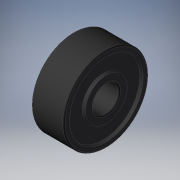
# Autodesk Inventor part: B624ZZ
Saved by Autodesk Inventor 2019 (Build 230136000, 136)
## iProperties
Created: 2024-10-07
Part Number: B624ZZ
Material: Generic
Catalog Web Link: www.cadenas.de
Description: B6 _ _ ZZ, B6 _ _ AZZ, SB6 _ _ ZZ, SB6 _ _ AZZ, BR _ _ ZZ, SBR _ _ ZZ-Small Ball Bearings - Double Shield Type
Vendor: MISUMI
Document SubType Name: Modeling
Designer: psAdmin
Manufacturer: MISUMI
Mass: 0.528594 g
Surface Area: 5.56418 cm^2
Volume: 0.528594 cm^3
Density: 1 g/cm^3
Appearance: PSOLRGB-175-175-175
Category: PARTsolutions
Company: MISUMI
Title: B624ZZ
Author: Cadenas PARTsolutions
Comments: Small Ball Bearings - Double Shield Type
PSOL_IDENT_0: {$CADENAS_DATA/23d-libs/misumi/metric/12_bearing_holders/sb685zz.prj},218 {VTYP=3D},{NB=B624ZZ},{LIN
PSOL_IDENT_1: A=B624ZZ},{NN=B6 _ _ ZZ, B6 _ _ AZZ, SB6 _ _ ZZ, SB6 _ _ AZZ, BR _ _ ZZ, SBR _ _ ZZ},{DATE=30.06.202
PSOL_IDENT_2: 1 12:59:24},{GEOMDATE=23.07.2013 00:00:00},{VERSION=},{LINEID=60},{WBVAR=MAT},{WBNUMERIC=}  {NB=B624
PSOL_IDENT_3: ZZ},{LINA=B624ZZ},{KT=DUMMY},{PN=B624ZZ},{MAT=},{BN=624ZZ},{DD=4.0},{A=3.9530},{BB=0.850},{C=1.200},
PSOL_IDENT_4: {D=13},{B=5.0},{RR=0.20},{CR=1310},{COR=490},{CRS=1310},{CRSS=1106},{CORS=490},{CORSS=390},{DS=5.60}
PSOL_IDENT_5: ,{DDHH=11.40},{R=0.20},{MASS=3.2},{X=0},{BN2=B624ZZ}
NB: B624ZZ
NN: B6 _ _ ZZ, B6 _ _ AZZ, SB6 _ _ ZZ, SB6 _ _ AZZ, BR _ _ ZZ, SBR _ _ ZZ
NT: Small Ball Bearings - Double Shield Type
NBSYN: $PN.
LINA: B624ZZ
CATALOG: Misumi
PN: B624ZZ
MAT: 52100 Bearing Steel
BN: 624ZZ
DD: 4
D: 13
B: 5
RR: 0.2
CR: 1310
COR: 490
DS: 5.6
DDHH: 11.4
R: 0.2
MASS: 3.2
X: 0
SUPPLIER: MISUMI
ARTICLENO: B624ZZ
BOMINFO: B624ZZ
CREATOR: CADENAS GmbH
Autodesk Inventor part; units mm, degrees
sketch "Sketch_1" plane through (0, 0, 0) normal (0, 0, 1) x (1, 0, 0)
  line L0 (4.8, 0) -> (0.2, 0)
  arc A0 (0, 2.2) -> (0.2, 2) centre (0.2, 2.2) ccw
  line L1 (0.2, 2) -> (4.8, 2)
  arc A1 (4.8, 2) -> (5, 2.2) centre (4.8, 2.2) ccw
  line L2 (5, 2.2) -> (5, 3.2)
  line L3 (5, 3.2) -> (4.4765, 3.2)
  line L4 (4.4765, 3.2) -> (4.4765, 5.65)
  line L5 (4.4765, 5.65) -> (5, 5.65)
  line L6 (5, 5.65) -> (5, 6.3)
  arc A2 (5, 6.3) -> (4.8, 6.5) centre (4.8, 6.3) ccw
  line L7 (4.8, 6.5) -> (0.2, 6.5)
  arc A3 (0.2, 6.5) -> (0, 6.3) centre (0.2, 6.3) ccw
  line L8 (0, 6.3) -> (0, 5.65)
  line L9 (0, 5.65) -> (0.5235, 5.65)
  line L10 (0.5235, 5.65) -> (0.5235, 3.2)
  line L11 (0.5235, 3.2) -> (0, 3.2)
  line L12 (0, 3.2) -> (0, 2.2)
  constraints: 26 end point, 8 point on circle, 4 centre point
revolve "Revolution1" add sketch "Sketch_1" angle 360 about axis through (4.8, 0, 0) along (1, 0, 0)
ref_plane "to_housing_XY" through (0, 0, 0) normal (1, 0, 0) x (0, 0, -1)
ref_plane "to_housing_YZ" through (0, 0, 0) normal (0, 0, -1) x (0, 1, 0)
ref_plane "to_housing_ZX" through (0, 0, 0) normal (0, 1, 0) x (1, 0, 0)
ref_plane "to_housing_center_XY" through (2.5, 0, 0) normal (1, 0, 0) x (0, 0, -1)
ref_plane "to_housing_center_YZ" through (2.5, 0, 0) normal (0, 0, -1) x (0, 1, 0)
ref_plane "to_housing_center_ZX" through (2.5, 0, 0) normal (0, 1, 0) x (1, 0, 0)
body "Solid1"
